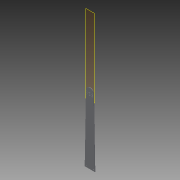
# Autodesk Inventor part: octoBotoStemSectD_v01
Saved by Autodesk Inventor 2013 (Build 170138000, 138)
## iProperties
Created: 2014-08-27
Part Number: octoBotoStemSectD_v01
Material: Generic
Document SubType Name: Modeling
Designer: Nano
Density: 1 g/cm^3
Author: Nano
Autodesk Inventor part; units mm, degrees
ref_plane "YZ Plane" through (0, 0, 0) normal (1, 0, 0) x (0, 1, 0)
ref_plane "XZ Plane" through (0, 0, 0) normal (0, 1, 0) x (-1, 0, 0)
ref_plane "XY Plane" through (0, 0, 0) normal (0, 0, 1) x (1, 0, 0)
ref_plane "Work Plane1" through (0, 0, 0) normal (0, 0, 1) x (1, 0, 0)
sketch "Sketch1" plane through (0, 0, 0) normal (0, 0, 1) x (1, 0, 0)
  circle A0 centre (15.2714, 289.6793) radius 1.651 projected
  circle A1 centre (2.5714, 289.6793) radius 1.651 projected
  circle A2 centre (-10.1286, 289.6793) radius 1.651 projected
  circle A3 centre (15.2714, 283.3293) radius 1.651 projected
  circle A4 centre (2.5714, 283.3293) radius 1.651 projected
  circle A5 centre (-10.1286, 283.3293) radius 1.651 projected
  circle A6 centre (15.2714, 276.9793) radius 1.651 projected
  circle A7 centre (2.5714, 276.9793) radius 1.651 projected
  circle A8 centre (-10.1286, 276.9793) radius 1.651 projected
  circle A9 centre (15.2714, 270.6293) radius 1.651 projected
  circle A10 centre (2.5714, 270.6293) radius 1.651 projected
  circle A11 centre (-10.1286, 270.6293) radius 1.651 projected
  circle A12 centre (15.2714, 264.2793) radius 1.651 projected
  circle A13 centre (2.5714, 264.2793) radius 1.651 projected
  circle A14 centre (-10.1286, 264.2793) radius 1.651 projected
  circle A15 centre (-16.4786, 264.2793) radius 1.651 projected
  circle A16 centre (-3.7786, 264.2793) radius 1.651 projected
  circle A17 centre (8.9214, 264.2793) radius 1.651 projected
  circle A18 centre (-16.4786, 270.6293) radius 1.651 projected
  circle A19 centre (-3.7786, 270.6293) radius 1.651 projected
  circle A20 centre (8.9214, 270.6293) radius 1.651 projected
  circle A21 centre (-16.4786, 276.9793) radius 1.651 projected
  circle A22 centre (-3.7786, 276.9793) radius 1.651 projected
  circle A23 centre (8.9214, 276.9793) radius 1.651 projected
  circle A24 centre (-16.4786, 283.3293) radius 1.651 projected
  circle A25 centre (-3.7786, 283.3293) radius 1.651 projected
  circle A26 centre (8.9214, 283.3293) radius 1.651 projected
  circle A27 centre (-16.4786, 289.6793) radius 1.651 projected
  circle A28 centre (-3.7786, 289.6793) radius 1.651 projected
  circle A29 centre (8.9214, 289.6793) radius 1.651 projected
  circle A30 centre (25.4672, -253.1178) radius 1.651 projected
  circle A31 centre (19.1172, -253.1178) radius 1.651 projected
  circle A32 centre (12.7672, -253.1178) radius 1.651 projected
  circle A33 centre (6.4172, -253.1178) radius 1.651 projected
  circle A34 centre (0.0672, -253.1178) radius 1.651 projected
  circle A35 centre (-6.2828, -253.1178) radius 1.651 projected
  circle A36 centre (-12.6328, -253.1178) radius 1.651 projected
  circle A37 centre (-18.9828, -253.1178) radius 1.651 projected
  circle A38 centre (-25.3328, -253.1178) radius 1.651 projected
  circle A39 centre (25.4672, -259.4678) radius 1.651 projected
  circle A40 centre (19.1172, -259.4678) radius 1.651 projected
  circle A41 centre (12.7672, -259.4678) radius 1.651 projected
  circle A42 centre (6.4172, -259.4678) radius 1.651 projected
  circle A43 centre (0.0672, -259.4678) radius 1.651 projected
  circle A44 centre (-6.2828, -259.4678) radius 1.651 projected
  circle A45 centre (-12.6328, -259.4678) radius 1.651 projected
  circle A46 centre (-18.9828, -259.4678) radius 1.651 projected
  circle A47 centre (-25.3328, -259.4678) radius 1.651 projected
  circle A48 centre (25.4672, -265.8178) radius 1.651 projected
  circle A49 centre (19.1172, -265.8178) radius 1.651 projected
  circle A50 centre (12.7672, -265.8178) radius 1.651 projected
  circle A51 centre (6.4172, -265.8178) radius 1.651 projected
  circle A52 centre (0.0672, -265.8178) radius 1.651 projected
  circle A53 centre (-6.2828, -265.8178) radius 1.651 projected
  circle A54 centre (-12.6328, -265.8178) radius 1.651 projected
  circle A55 centre (-18.9828, -265.8178) radius 1.651 projected
  circle A56 centre (-25.3328, -265.8178) radius 1.651 projected
  circle A57 centre (25.4672, -272.1678) radius 1.651 projected
  circle A58 centre (19.1172, -272.1678) radius 1.651 projected
  circle A59 centre (12.7672, -272.1678) radius 1.651 projected
  circle A60 centre (6.4172, -272.1678) radius 1.651 projected
  circle A61 centre (0.0672, -272.1678) radius 1.651 projected
  circle A62 centre (-6.2828, -272.1678) radius 1.651 projected
  circle A63 centre (-12.6328, -272.1678) radius 1.651 projected
  circle A64 centre (-18.9828, -272.1678) radius 1.651 projected
  circle A65 centre (-25.3328, -272.1678) radius 1.651 projected
  circle A66 centre (25.4672, -278.5178) radius 1.651 projected
  circle A67 centre (19.1172, -278.5178) radius 1.651 projected
  circle A68 centre (12.7672, -278.5178) radius 1.651 projected
  circle A69 centre (6.4172, -278.5178) radius 1.651 projected
  circle A70 centre (0.0672, -278.5178) radius 1.651 projected
  circle A71 centre (-6.2828, -278.5178) radius 1.651 projected
  circle A72 centre (-12.6328, -278.5178) radius 1.651 projected
  circle A73 centre (-18.9828, -278.5178) radius 1.651 projected
  circle A74 centre (-25.3328, -278.5178) radius 1.651 projected
  arc A75 (22.3491, 290.0954) -> (-22.3491, 290.0954) centre (0, 289.6793) ccw projected
  line L0 (-22.3491, 290.0954) -> (-33.0532, -284.8678) projected
  line L1 (-33.0532, -284.8678) -> (33.0532, -284.8678) projected
  line L2 (33.0532, -284.8678) -> (22.3491, 290.0954) projected
  arc A76 (32.4033, -249.9589) -> (-32.4033, -249.9589) centre (0, -250.5622) ccw
  line L3 (-32.4033, -249.9589) -> (-42.9236, -815.0533)
  line L4 (-42.9236, -815.0533) -> (42.9236, -815.0533)
  line L5 (42.9236, -815.0533) -> (32.4033, -249.9589)
  line L6 (-32.4033, -218.1533) -> (33.9104, -218.1533) construction
  point P0 (0, 0)
  dimension "d0" = 596.9
  constraints: 8 end point, 3 tangent, 2 collinear, 2 point on circle, 1 centre point, 1 horizontal
  measures "d0" distance between parallel lines of L4 L6
extrude "Extrusion1" add sketch "Sketch1" along normal blind 3.175 contours L2 L1 L0 A76 | L5 L4 L3 L1
sketch "Sketch2" plane through (0, 0, 3.175) normal (0, 0, 1) x (1, 0, 0)
  line L0 (-42.9236, -815.0533) -> (42.9236, -815.0533) projected
  circle A0 centre (-30.2236, -802.3533) radius 3.175
  line L1 (0, -815.0533) -> (0, -733.814) construction
  circle A1 centre (30.2236, -802.3533) radius 3.175
  point P0 (0, 0)
  dimension "d4" = 6.35
  dimension "d5" = 12.7
  dimension "d6" = 12.7
  constraints: 2 centre point, 2 end point, 1 symmetric about line, 1 other
  measures "d4" diameter of A0
  measures "d5" distance from line of L0 A0.centre
  measures "d6" horizontal distance of L0.start A0.centre
extrude "Extrusion2" cut sketch "Sketch2" against normal through all
body "Solid1"
